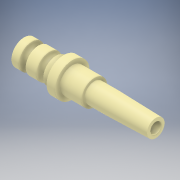
# Autodesk Inventor part: Connection
Saved by Autodesk Inventor 2017 (Build 210142000, 142)
## iProperties
Created: 2023-05-03
Part Number: Connection
Material: Nylon 6/6
Document SubType Name: Modeling
Designer: Vinicius Silva
Density: 1.13 g/cm^3
Appearance: Nylon 6
Author: Vinicius Silva
Autodesk Inventor part; units mm, degrees
ref_plane "YZ Plane" through (0, 0, 0) normal (1, 0, 0) x (0, 1, 0)
ref_plane "XZ Plane" through (0, 0, 0) normal (0, 1, 0) x (-1, 0, 0)
sketch "Sketch1" plane through (0, 0, 0) normal (0, 1, 0) x (-1, 0, 0)
  line L0 (0, 0) -> (30, 0)
  line L1 (30, 0) -> (30, -2.9)
  line L2 (30, -2.9) -> (14, -2.9)
  line L3 (0, 0) -> (0, -2)
  line L4 (0, -2) -> (10, -2.25)
  line L5 (14, -2.9) -> (14, -2.25)
  line L6 (10, -2.25) -> (14, -2.25)
  dimension "d0" = 30
  dimension "d1" = 2.9
  dimension "d2" = 16
  dimension "d3" = 2
  dimension "d5" = 4.5
  dimension "d6" = 10
  dimension "d20" = 4
  constraints: 14 end point, 3 vertical, 2 horizontal, 1 parallel
  measures "d0" distance of L0.start L0.end
  measures "d1" distance of L0.end L1.end
  measures "d2" distance of L1.end L2.end
  measures "d3" distance of L0.start L3.end
  measures "d5" diameter of L4.end L0
  measures "d6" horizontal distance of L3.end L4.end
  measures "d20" distance of L4.end L5.end
revolve "Revolution1" add sketch "Sketch1" angle 360 about axis through (0, 0, 0) along (-1, 0, 0)
sketch "Sketch2" plane through (0, 0, 0) normal (0, 0, 1) x (1, 0, 0)
  line L0 (-14, -2.9) -> (-14, 2.9) construction
  line L1 (-30, -2.9) -> (-30, 2.9) construction
  line L2 (-30, 2.9) -> (-14, 2.9) projected
  line L3 (-30, -2.9) -> (-30, 2.9) projected
  line L4 (-30, 0) -> (0, 0)
  line L5 (-19, 1.9) -> (-19, 3.9)
  line L6 (-19, 3.9) -> (-21, 3.9)
  line L7 (-21, 3.9) -> (-21, 1.9)
  line L8 (-21, 1.9) -> (-19, 1.9)
  line L9 (-30, 2.9) -> (-14, 2.9) projected
  line L10 (-19, 1.9) -> (-21, 3.9) construction
  line L11 (-19, 3.9) -> (-21, 1.9) construction
  line L12 (-30, 2.9) -> (-14, 2.9) projected
  point P0 (-20, 2.9)
  dimension "d39" = 2
  dimension "d40" = 1
  dimension "d42" = 5
  constraints: 14 end point, 3 midpoint, 2 parallel, 2 perpendicular, 1 horizontal, 1 point on line
  measures "d39" distance of L5.end L6.end
  measures "d40" distance from line of L6 point (-20, 2.9)
  measures "d42" distance from line of L5 L2.end
revolve "Revolution2" add sketch "Sketch2" angle 360 about axis through (-30, 0, 0) along (1, 0, 0)
sketch "Sketch4" plane through (0, 0, 0) normal (1, 0, 0) x (0, 0, -1)
  circle A0 centre (0, 0) radius 1.25
  dimension "d14" = 2.5
  constraints: 1 centre point, 1 coincident
  measures "d14" diameter of A0
extrude "Extrusion1" cut sketch "Sketch4" against normal through all
ref_plane "Work Plane1" through (-22, 0, 2.9) normal (0, 0, 1) x (1, 0, 0)
sketch "Sketch3" plane through (0, 0, 0) normal (0, 0, 1) x (1, 0, 0)
  line L0 (-30, -2.9) -> (-30, 2.9) projected
  line L1 (-30, 0) -> (0, 0)
  line L2 (-27.5, 3.2) -> (-27.5, 2.6) construction
  line L3 (-30, 2.9) -> (-21, 2.9) projected
  line L4 (-30, 2.9) -> (-21, 2.9) projected
  line L5 (-28.25, 3.2) -> (-28.25, 2.6)
  line L6 (-26.75, 2.6) -> (-26.75, 3.2)
  arc A0 (-26.75, 3.2) -> (-28.25, 3.2) centre (-27.5, 3.2) ccw
  arc A1 (-28.25, 2.6) -> (-26.75, 2.6) centre (-27.5, 2.6) ccw
  line L7 (-23.5, 3.2) -> (-23.5, 2.6) construction
  line L8 (-24.25, 3.2) -> (-24.25, 2.6)
  line L9 (-22.75, 2.6) -> (-22.75, 3.2)
  arc A2 (-22.75, 3.2) -> (-24.25, 3.2) centre (-23.5, 3.2) ccw
  arc A3 (-24.25, 2.6) -> (-22.75, 2.6) centre (-23.5, 2.6) ccw
  point P0 (-27.5, 2.9)
  point P1 (-23.5, 2.9)
  dimension "d28" = 1.5
  dimension "d29" = 0.3
  dimension "d30" = 2.5
  dimension "d34" = 4
  constraints: 18 end point, 8 point on circle, 4 centre point, 4 tangent, 2 horizontal, 2 midpoint, 1 parallel, 1 perpendicular, 14 other
  measures "d28" diameter of A1
  measures "d29" distance of point (-27.5, 2.9) L2.end
  measures "d30" distance between parallel lines of L0 L2
  measures "d34" distance of L5.start L8.start
revolve "Revolution5" cut sketch "Sketch3" angle 360 about axis through (-30, 0, 0) along (1, 0, 0)
body "Solid1"
